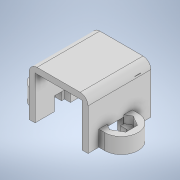
# Autodesk Inventor part: mocowanie_silnik
Saved by Autodesk Inventor 2020.3 (Build 243373000, 373)
## iProperties
Created: 2021-05-10
Part Number: mocowanie_silnik
Material: Ogólny
Document SubType Name: Modeling
Designer: patry
Density: 1 g/cm^3
Appearance: Domyślna
Author: patry
Autodesk Inventor part; units mm, degrees
ref_plane "YZ Plane" through (0, 0, 0) normal (1, 0, 0) x (0, 1, 0)
ref_plane "XZ Plane" through (0, 0, 0) normal (0, 1, 0) x (-1, 0, 0)
ref_plane "XY Plane" through (0, 0, 0) normal (0, 0, 1) x (1, 0, 0)
sketch "Szkic1" plane through (0, 0, 0) normal (0, 0, 1) x (1, 0, 0)
  line L0 (0, 0) -> (15, 0)
  line L1 (15, 0) -> (15, 11.5)
  line L2 (15, 11.5) -> (0, 11.5)
  line L3 (0, 11.5) -> (0, 0)
  line L4 (1.5, 1.5) -> (13.5, 1.5)
  line L5 (13.5, 1.5) -> (13.5, 10)
  line L6 (13.5, 10) -> (1.5, 10)
  line L7 (1.5, 10) -> (1.5, 1.5)
  line L8 (1.5, 1.5) -> (1.5, 0)
  line L9 (13.5, 1.5) -> (13.5, 0)
  line L10 (0, 0) -> (15, 0)
  line L11 (15, 0) -> (15, -1)
  line L12 (15, -1) -> (0, -1)
  line L13 (0, -1) -> (0, 0)
  line L14 (13.5, 0) -> (13.5, -1)
  line L15 (1.5, 0) -> (1.5, -1)
  dimension "d0" = 15
  dimension "d1" = 11.5
  dimension "d2" = 1.5
  dimension "d3" = 1
  constraints: 32 end point, 6 parallel, 6 perpendicular, 4 point on line, 2 horizontal, 1 vertical, 3 other
  measures "d0" distance of L2.end L1.end
  measures "d1" distance of L1.end L0.end
  measures "d2" distance between parallel lines of L3 L7
  measures "d3" distance of L10.end L11.end
extrude "Wyciągnięcie proste1" add sketch "Szkic1" along normal blind 20 contours L3 L2 L1 L0 L9 L5 L6 L7 L8 | L0 L15 L12 L13 | L0 L11 L12 L14
fillet "Zaokrąglenie1" radius 2 2 edges at (15, 11.5, 10) (0, 11.5, 10)
sketch "Szkic2" plane through (13.5, -1, 0) normal (0, -1, 0) x (1, 0, 0)
  line L0 (-13.5, 0) -> (-13.5, 20) projected
  line L1 (1.5, 0) -> (1.5, 20) projected
  line L2 (0, 0) -> (1.5, 0) projected
  circle A0 centre (3, 13) radius 1.25
  circle A1 centre (-15, 13) radius 1.25
  circle A2 centre (3, 13) radius 4.25
  circle A3 centre (-15, 13) radius 4.25
  line L3 (3, 8.75) -> (1.5, 8.75)
  line L4 (-15, 8.75) -> (-13.5, 8.75)
  line L5 (3, 17.25) -> (1.5, 17.25)
  line L6 (-15, 17.25) -> (-13.5, 17.25)
  dimension "d7" = 1.5
  dimension "d8" = 1.5
  dimension "d9" = 13
  dimension "d10" = 2.5
  dimension "d11" = 2.5
  dimension "d12" = 8.5
  dimension "d13" = 8.5
  constraints: 8 end point, 8 point on line, 4 centre point, 4 coincident, 4 point on circle, 1 horizontal, 1 horizontal alignment, 1 perpendicular, 1 tangent
  measures "d7" distance from line of L0 point (-15, 13)
  measures "d8" distance from line of L1 point (3, 13)
  measures "d9" distance from line of L2 point (3, 13)
  measures "d10" diameter of A0
  measures "d11" diameter of A1
  measures "d12" diameter of A2
  measures "d13" diameter of A3
extrude "Wyciągnięcie proste2" add sketch "Szkic2" against normal blind 2 contours L4 A3 L0 | A3 L0 | A3 L6 L0 | L1 A2 L3 | L1 A2 | L1 L5 A2 picked at (-15.3893, 9.7942) picked at (6.2145, 12.6848)
sketch "Szkic3" plane through (0, -1, 0) normal (0, -1, 0) x (1, 0, 0)
  line L0 (1.5, 0) -> (1.5, 20) projected
  line L1 (1.5, 11) -> (0, 11)
  line L2 (0, 11) -> (0, 15)
  line L3 (0, 15) -> (1.5, 15)
  line L4 (1.5, 15) -> (1.5, 11)
  circle A0 centre (-1.5, 13) radius 1.25 projected
  line L5 (0, 0) -> (0, 20) projected
  line L6 (-1.5, 11.75) -> (0, 11.75)
  line L7 (0, 11.75) -> (0, 14.25)
  line L8 (0, 14.25) -> (-1.5, 14.25)
  line L9 (-1.5, 14.25) -> (-1.5, 11.75)
  line L10 (13.5, 0) -> (13.5, 20) projected
  line L11 (13.5, 11) -> (15, 11)
  line L12 (15, 11) -> (15, 15)
  line L13 (15, 15) -> (13.5, 15)
  line L14 (13.5, 15) -> (13.5, 11)
  circle A1 centre (16.5, 13) radius 1.25 projected
  line L15 (16.5, 11.75) -> (15, 11.75)
  line L16 (15, 11.75) -> (15, 14.25)
  line L17 (15, 14.25) -> (16.5, 14.25)
  line L18 (16.5, 14.25) -> (16.5, 11.75)
  dimension "d16" = 1.5
  dimension "d17" = 4
  dimension "d18" = 2
  dimension "d19" = 1.5
  dimension "d20" = 4
  constraints: 32 end point, 8 parallel, 4 horizontal, 4 perpendicular, 4 point on line, 4 other
  measures "d16" distance of L2.end L3.end
  measures "d17" distance of L1.end L2.end
  measures "d18" distance from line of L3 point (-1.5, 13)
  measures "d19" distance of L13.end L12.end
  measures "d20" distance of L12.end L11.end
extrude "Wyciągnięcie proste3" cut sketch "Szkic3" against normal blind 3.5 contours L1 L2 L3 L0 | L6 A0 L8 L2 | L10 L13 L12 L11 | L12 L17 A1 L15 | L18 A1 | A1 L18
sketch "Szkic4" plane through (13.5, 1, 0) normal (0, 1, 0) x (1, 0, 0)
  arc A0 (-15, -11.75) -> (-15, -14.25) centre (-15, -13) ccw projected
  arc A1 (3, -14.25) -> (3, -11.75) centre (3, -13) ccw projected
  arc A2 (3, -17.25) -> (3, -8.75) centre (3, -13) ccw projected
  line L0 (3, -16) -> (0.4019, -14.5)
  line L1 (0.4019, -14.5) -> (0.4019, -11.5)
  line L2 (0.4019, -11.5) -> (3, -10)
  line L3 (3, -10) -> (5.5981, -11.5)
  line L4 (5.5981, -11.5) -> (5.5981, -14.5)
  line L5 (5.5981, -14.5) -> (3, -16)
  line L6 (-15, -16) -> (-17.5981, -14.5)
  line L7 (-17.5981, -14.5) -> (-17.5981, -11.5)
  line L8 (-17.5981, -11.5) -> (-15, -10)
  line L9 (-15, -10) -> (-12.4019, -11.5)
  line L10 (-12.4019, -11.5) -> (-12.4019, -14.5)
  line L11 (-12.4019, -14.5) -> (-15, -16)
  line L12 (1.5, -11.75) -> (3, -11.75) projected
  arc A3 (3, -14.25) -> (3, -11.75) centre (3, -13) ccw projected
  line L13 (3, -14.25) -> (1.5, -14.25) projected
  line L14 (1.5, -15) -> (1.5, -14.25) projected
  line L15 (1.5, -17.25) -> (1.5, -15) projected
  line L16 (1.5, -17.25) -> (3, -17.25) projected
  arc A4 (3, -17.25) -> (3, -8.75) centre (3, -13) ccw projected
  line L17 (3, -8.75) -> (1.5, -8.75) projected
  line L18 (1.5, -11) -> (1.5, -8.75) projected
  line L19 (1.5, -11.75) -> (1.5, -11) projected
  line L20 (-15, -11.75) -> (-13.5, -11.75) projected
  line L21 (-13.5, -11) -> (-13.5, -11.75) projected
  line L22 (-13.5, -8.75) -> (-13.5, -11) projected
  line L23 (-13.5, -8.75) -> (-15, -8.75) projected
  arc A5 (-15, -8.75) -> (-15, -17.25) centre (-15, -13) ccw projected
  line L24 (-15, -17.25) -> (-13.5, -17.25) projected
  line L25 (-13.5, -15) -> (-13.5, -17.25) projected
  line L26 (-13.5, -14.25) -> (-13.5, -15) projected
  line L27 (-13.5, -14.25) -> (-15, -14.25) projected
  arc A6 (-15, -11.75) -> (-15, -14.25) centre (-15, -13) ccw projected
  point P0 (-13.5, 0)
  point P1 (-13.5, -10.866)
  point P2 (-13.5, -15.134)
  point P3 (1.5, -15.134)
  point P4 (1.5, -10.866)
  dimension "d23" = 6
  constraints: 24 end point, 2 coincident, 26 other
  measures "d23" distance of L2.end L0.start
extrude "Wyciągnięcie proste4" add sketch "Szkic4" along normal blind 2 contours L9 L8 L7 L6 L11 L25 L24 A5 L23 L22 | L0 L5 L4 L3 L2 L18 L17 A2 L16 L15
sketch "Szkic5" plane through (1.5, 10, 0) normal (0, -1, 0) x (1, 0, 0)
  arc A0 (-3, 14.25) -> (-3, 11.75) centre (-3, 13) ccw projected
  arc A1 (15, 11.75) -> (15, 14.25) centre (15, 13) ccw projected
  line L0 (3.4539, 6.5) -> (13.4539, 6.5)
  line L1 (13.4539, 6.5) -> (13.4539, 8)
  line L2 (13.4539, 8) -> (3.4539, 8)
  line L3 (3.4539, 8) -> (3.4539, 6.5)
  point P0 (-1.5, 0)
  dimension "d26" = 10
  dimension "d27" = 1.5
  dimension "d28" = 5
  constraints: 8 end point, 2 parallel, 1 horizontal, 1 perpendicular
  measures "d26" distance of L2.end L1.end
  measures "d27" distance of L1.end L0.end
  measures "d28" distance from line of A1.centre L2
extrude "Wyciągnięcie proste5" add sketch "Szkic5" along normal blind 2
sketch "Szkic6" plane through (2, 11.5, 0) normal (0, 1, 0) x (1, 0, 0)
  line L0 (-2, 0) -> (0, 0) projected
  line L1 (13, 0) -> (13, -8.75) projected
  line L2 (-2, 0) -> (13, 0)
  line L3 (13, 0) -> (13, -4)
  line L4 (13, -4) -> (-2, -4)
  line L5 (-2, -4) -> (-2, 0)
  dimension "d31" = 4
  constraints: 8 end point, 2 parallel, 1 horizontal, 1 perpendicular, 1 point on line
  measures "d31" distance of L2.end L3.end
extrude "Wyciągnięcie proste6" cut sketch "Szkic6" against normal through all
